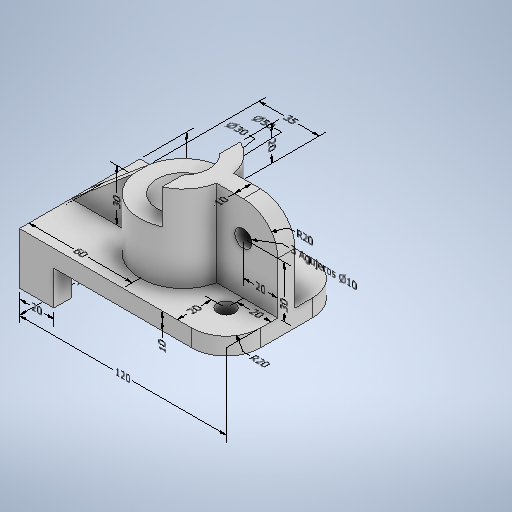
# Autodesk Inventor part: Pieza1
Saved by Autodesk Inventor 2027.1 (Build 311270010, 270A)
## iProperties
Created: 2026-09-20
Part Number: Pieza1
Material: Genérico
Document SubType Name: Modeling
Designer: atlas
Density: 1 g/cm^3
Appearance: Valor por defecto
Author: atlas
Autodesk Inventor part; units mm, degrees
ref_plane "YZ Plane" through (0, 0, 0) normal (1, 0, 0) x (0, 1, 0)
ref_plane "XZ Plane" through (0, 0, 0) normal (0, 1, 0) x (-1, 0, 0)
ref_plane "XY Plane" through (0, 0, 0) normal (0, 0, 1) x (1, 0, 0)
sketch "Boceto1" plane through (0, 0, 0) normal (0, 1, 0) x (-1, 0, 0)
  line L0 (20, 0) -> (120, 0)
  line L1 (120, 0) -> (120, -70)
  line L2 (120, -70) -> (20, -70)
  line L3 (0, -50) -> (0, -20)
  arc A0 (20, 0) -> (0, -20) centre (20, -20) ccw
  arc A1 (0, -50) -> (20, -70) centre (20, -50) ccw
  circle A2 centre (20, -20) radius 5
  circle A3 centre (20, -50) radius 5
  line L4 (120, -35) -> (60, -35)
  line L5 (120, -35) -> (180, -35) construction
  circle A4 centre (60, -35) radius 15
  circle A5 centre (60, -35) radius 25
  line L6 (120, -39.9519) -> (120, -29.9405)
  line L7 (120, -30) -> (155.5051, -30) construction
  line L8 (120, -40) -> (155.5051, -40) construction
  line L9 (120, -40) -> (84.4949, -40)
  line L10 (35.5051, -40) -> (0, -40)
  line L11 (120, -30) -> (84.4949, -30)
  line L12 (35.5051, -30) -> (0, -30)
  point P0 (0, 0)
  point P1 (0, -70)
  dimension "d0" = 120
  dimension "d1" = 70
  dimension "d2" = 20
  dimension "d3" = 20
  dimension "d4" = 10
  dimension "d5" = 10
  dimension "d6" = 60
  dimension "d7" = 180
  dimension "d8" = 30
  dimension "d9" = 50
  constraints: 26 end point, 9 point on line, 8 point on circle, 6 centre point, 5 horizontal, 4 coincident, 4 tangent, 2 parallel, 1 collinear, 1 midpoint, 1 perpendicular
  measures "d0" distance of L1.end point (0, -70)
  measures "d1" distance of L0.end L1.end
  measures "d2" radius of A0
  measures "d3" radius of A1
  measures "d4" diameter of A2
  measures "d5" diameter of A3
  measures "d6" distance of L4.start L4.end
  measures "d7" angle of L4 L5
  measures "d8" diameter of A4
  measures "d9" diameter of A5
extrude "Extrusión1" add sketch "Boceto1" along normal blind 10 contours L0 L1 L11 A5 L12 L3 A0 | L10 A5 L9 L1 L2 A1 L3
extrude "Extrusión2" add sketch "Boceto1" along normal blind 60 contours L12 A5 L10 L3 | L1 L4 A5 L11 | A5 | L1 L9 A5 L4
fillet "Empalme1" radius 20 1 edges at (0, 60, -35)
sketch "Boceto2" plane through (-120, 10, -30) normal (0, 0, 1) x (1, 0, 0)
  line L0 (35.5051, 0) -> (84.4949, 0) projected
  line L1 (35.5051, 0) -> (35.5051, 30)
  line L2 (0, 0) -> (100, 0) projected
  line L3 (35.5051, 30) -> (0, 0)
  line L4 (35.5051, 30) -> (70.5051, 30)
  line L5 (70.5051, 30) -> (70.5051, 50)
  line L6 (84.4949, 50) -> (35.5051, 50) projected
  line L7 (35.5051, 30) -> (35.5051, 50)
  line L8 (35.5051, 50) -> (0, 50)
  line L9 (0, 50) -> (0, 0)
  line L10 (70.5051, 30) -> (70.5051, 50)
  line L11 (84.4949, 50) -> (35.5051, 50) projected
  line L12 (35.5051, 50) -> (35.5051, 30)
  line L13 (0, 0) -> (35.5051, 30)
  line L14 (70.5051, 30) -> (35.5051, 30)
  line L15 (70.5051, 30) -> (70.5051, 50)
  line L16 (70.5051, 50) -> (0, 50)
  line L17 (0, 50) -> (0, 0)
  dimension "d17" = 30
  dimension "d18" = 35
  dimension "d19" = 20
  constraints: 28 end point, 7 perpendicular, 3 collinear, 2 vertical
  measures "d17" distance of L0.start L1.end
  measures "d18" distance of L1.end L4.end
  measures "d19" distance of L4.end L5.end
extrude "Extrusión4" cut sketch "Boceto2" along normal mid plane 60 contours L7 L6 L5 L4 | L3 L9 L8 L7
sketch "Boceto3" plane through (-35.5051, 10, -30) normal (0, 0, 1) x (1, 0, 0)
  line L0 (35.5051, 0) -> (35.5051, 30) projected
  line L1 (35.5051, 0) -> (15.5051, 0) projected
  line L2 (35.5051, 0) -> (15.5051, 0)
  line L3 (15.5051, 0) -> (15.5051, 30)
  circle A0 centre (15.5051, 30) radius 5
  point P0 (35.5051, -10)
  dimension "d25" = 10
  constraints: 4 end point, 1 centre point, 1 coincident, 1 collinear, 1 perpendicular
  measures "d25" diameter of A0
extrude "Extrusión5" cut sketch "Boceto3" against normal blind 60
sketch "Boceto4" plane through (0, 0, 0) normal (0, -1, 0) x (1, 0, 0)
  line L0 (-120, -30) -> (-120, 0) projected
  line L1 (-120, 0) -> (-100, 0)
  line L2 (-100, 0) -> (-100, -10)
  line L3 (-100, -10) -> (-120, -10)
  line L4 (-120, -10) -> (-120, 0)
  line L5 (-120, -60.1296) -> (-100, -60.1296)
  line L6 (-100, -60.1296) -> (-100, -70.1296)
  line L7 (-100, -70.1296) -> (-120, -70.1296)
  line L8 (-120, -70.1296) -> (-120, -60.1296)
  line L9 (-100, -10) -> (-100, -60.1296)
  line L10 (-120, -10) -> (-120, -60.1296)
  point P0 (0, 0)
  dimension "d28" = 20
  dimension "d29" = 10
  dimension "d30" = 20
  dimension "d31" = 10
  constraints: 20 end point, 4 parallel, 2 horizontal, 2 perpendicular, 1 collinear
  measures "d28" distance of L2.end L3.end
  measures "d29" distance of L1.end L2.end
  measures "d30" distance of L6.end L7.end
  measures "d31" distance of L5.end L6.end
extrude "Extrusión6" add sketch "Boceto4" along normal blind 10 contours L0 L3 L9 L5 L10
extrude "Extrusión7" add sketch "Boceto4" along normal blind 20 contours L0 L1 L2 L3 | L5 L6 L7 L8
